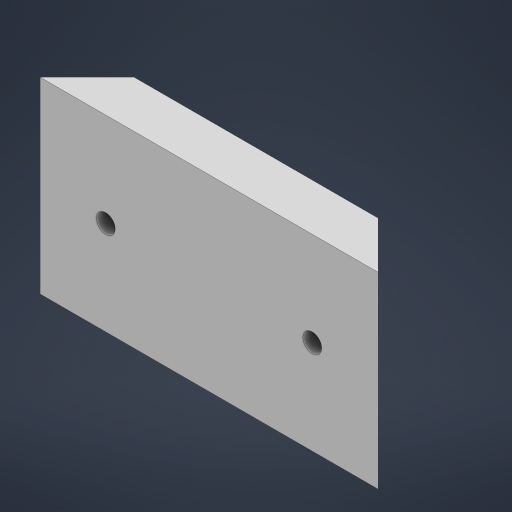
# Autodesk Inventor part: 3_inner_glider_carriage
Saved by Autodesk Inventor 2024 (Build 280153000, 153)
## iProperties
Created: 2023-05-23
Part Number: 3_inner_glider_carriage
Material: Generic
Document SubType Name: Modeling
Designer: aasmu
Density: 1 g/cm^3
Appearance: Default
ball_bearing_ID: 5.000 mm
ball_bearing_OD: 16.000 mm
ball_bearing_width: 5.000 mm
ball_bearing_mount_width: 5.000 mm
Author: aasmu
Autodesk Inventor part; units mm, degrees
ref_plane "YZ Plane" through (0, 0, 0) normal (1, 0, 0) x (0, 1, 0)
ref_plane "XZ Plane" through (0, 0, 0) normal (0, 1, 0) x (-1, 0, 0)
ref_plane "XY Plane" through (0, 0, 0) normal (0, 0, 1) x (1, 0, 0)
sketch "Sketch2" plane through (0, 0, 0) normal (1, 0, 0) x (0, 1, 0)
  line L0 (0, 0) -> (20, 0)
  line L1 (30, 10) -> (-10, 10)
  line L2 (-10, 20) -> (-10, 10)
  line L3 (30, 20) -> (30, 10)
  line L4 (20, 0) -> (30, 10)
  line L5 (0, 0) -> (-10, 10)
  line L6 (10, 0) -> (10, 7) construction
  circle A0 centre (10, 7) radius 2.5
  circle A1 centre (10, 7) radius 8 construction
  line L7 (-10, 20) -> (30, 20)
  arc A2 (18.4853, 10) -> (1.5147, 10) centre (10, 7) ccw
  point P0 (10, 10)
  point P1 (1.9377, 11)
  dimension "d12" = 10
  dimension "d15" = 45
  dimension "d16" = 20
  dimension "d17" = 7
  dimension "d18" = 5
  dimension "d19" = 16
  dimension "d21" = 10
  dimension "d22" = 9
  dimension "d55" = 11
  constraints: 16 end point, 3 centre point, 3 coincident, 3 perpendicular, 2 horizontal, 2 midpoint, 2 point on circle, 2 point on line, 2 vertical
  measures "d12" distance between parallel lines of L0 L1
  measures "d15" angle of L4 L0
  measures "d16" distance of L0.start L0.end
  measures "d17" distance of L6.start L6.end
  measures "d18" diameter of A0
  measures "d19" diameter of A1
  measures "d21" distance of L2.start L1.end
  measures "d22" radius of A2
extrude "Extrusion1" add sketch "Sketch2" along normal blind 5 contours L5 L1 L4 L0
extrude "Extrusion2" add sketch "Sketch2" against normal blind 6 contours L2 L7 L3 L1 A2
extrude "Extrusion3" add sketch "Sketch2" against normal blind 5 from surface at -6 contours L5 L1 L4 L0
extrude "Extrusion4" add sketch "Sketch2" along normal blind 23 contours L2 L7 L3 L1 A2 | A2 L1
extrude "Extrusion5" add sketch "Sketch2" against normal blind 23 from surface at -6 contours L2 L7 L3 L1 A2 | A2 L1
sketch "Sketch4" plane through (23, 30, 10) normal (0, 0, -1) x (-1, 0, 0)
  line L0 (52, -40) -> (52, 0) construction
  line L1 (52, -20) -> (0, -20) construction
  line L2 (0, 0) -> (0, -40) construction
  circle A0 centre (4, -20) radius 2
  line L3 (0, -40) -> (0, 0) construction
  circle A1 centre (48, -20) radius 2
  line L4 (52, 0) -> (52, -40) construction
  point P0 (23, -30)
  dimension "d39" = 4
  dimension "d40" = 4
  dimension "d41" = 4
  dimension "d42" = 4
  constraints: 4 midpoint, 2 centre point, 2 end point, 2 point on line
  measures "d39" distance of point (0, -20) A0.centre
  measures "d40" diameter of A0
  measures "d41" diameter of A1
  measures "d42" distance of point (52, -20) A1.centre
hole "Hole1" at (19, 10, 10) at (-25, 10, 10) direction (0, 0, 1) diameter 4 end through all counterbore diameter 6 counterbore depth 2
sketch "Sketch5" plane through (-6, 30, 10) normal (0, 1, 0) x (1, 0, 0)
  line L0 (-23, -10) -> (-23, 0) projected
  line L1 (-23, 0) -> (-33, -10)
  line L2 (-33, -10) -> (-23, -10)
  line L3 (-23, -10) -> (29, -10) projected
  line L4 (29, -10) -> (39, -10)
  line L5 (29, 0) -> (29, -10) projected
  line L6 (39, -10) -> (29, 0)
  point P0 (6, 10)
  dimension "d51" = 45
  dimension "d52" = 45
  constraints: 8 end point, 2 horizontal
  measures "d51" angle of L0 L1
  measures "d52" angle of L4 L6
extrude "Extrusion6" add sketch "Sketch5" against normal up to surface (40 mm away)
equation "\"d18\" = ball_bearing_ID"
equation "\"d19\" = ball_bearing_OD"
equation "\"d33\" = d29"
equation "\"d39\" = screw_size"
equation "\"d40\" = screw_size"
equation "\"d41\" = screw_size"
equation "\"d42\" = screw_size"
equation "\"d43\" = screw_size"
equation "\"ball_bearing_ID\" = 5"
equation "\"ball_bearing_OD\" = 16"
equation "\"ball_bearing_width\" = 5"
equation "\"screw_size\" = 4"
equation "\"d29\" = 23"
body "Solid1"
